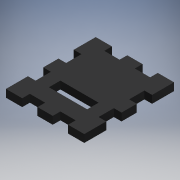
# Autodesk Inventor part: right
Saved by Autodesk Inventor 2019 (Build 230136000, 136)
## iProperties
Created: 2018-06-06
Part Number: right
Material: PBT Plastic Black
Document SubType Name: Modeling
Designer: stra92745
Density: 1.31 g/cm^3
Appearance: Smooth - White
Author: stra92745
Autodesk Inventor part; units mm, degrees
ref_plane "YZ Plane" through (0, 0, 0) normal (1, 0, 0) x (0, 1, 0)
ref_plane "XZ Plane" through (0, 0, 0) normal (0, 1, 0) x (-1, 0, 0)
ref_plane "XY Plane" through (0, 0, 0) normal (0, 0, 1) x (1, 0, 0)
sketch "Sketch1" plane through (0, 0, 0) normal (0, 1, 0) x (-1, 0, 0)
  line L0 (0, 0) -> (-41, 0)
  line L1 (-41, 0) -> (-41, -47)
  line L2 (-41, -47) -> (0, -47)
  line L3 (0, -47) -> (0, 0)
  line L4 (-10.5, -18) -> (-30.5, -18)
  line L5 (-30.5, -18) -> (-30.5, -12)
  line L6 (-30.5, -12) -> (-10.5, -12)
  line L7 (-10.5, -12) -> (-10.5, -18)
  dimension "d0" = 41
  dimension "d1" = 47
  dimension "d2" = 20
  dimension "d3" = 6
  dimension "d4" = 10.5
  dimension "d5" = 12
  constraints: 16 end point, 4 parallel, 2 horizontal, 2 perpendicular
  measures "d0" distance of L2.end L1.end
  measures "d1" distance of L1.end L0.end
  measures "d2" distance of L4.start L4.end
  measures "d3" distance of L4.end L5.end
  measures "d4" distance between parallel lines of L7 L3
  measures "d5" distance between parallel lines of L0 L6
extrude "Extrusion1" add sketch "Sketch1" along normal blind 4
sketch "Sketch2" plane through (0, 4, 0) normal (0, 1, 0) x (1, 0, 0)
  line L0 (41, 47) -> (0, 47) construction
  line L1 (0, 47) -> (0, 0) construction
  line L2 (0, 0) -> (41, 0) construction
  line L3 (41, 0) -> (41, 47) construction
  line L4 (4, 4) -> (4, 43) construction
  line L5 (4, 43) -> (37, 43) construction
  line L6 (37, 43) -> (37, 4) construction
  line L7 (37, 4) -> (4, 4) construction
  line L8 (0, 35.5) -> (4, 35.5)
  line L9 (4, 35.5) -> (4, 27.5)
  line L10 (4, 27.5) -> (0, 27.5)
  line L11 (0, 35.5) -> (0, 27.5)
  line L12 (0, 23.5) -> (41, 23.5) construction
  line L13 (20.5, 0) -> (20.5, 47) construction
  line L14 (41, 47) -> (0, 47) construction
  line L15 (8.5, 47) -> (8.5, 43)
  line L16 (8.5, 43) -> (16.5, 43)
  line L17 (16.5, 43) -> (16.5, 47)
  line L18 (16.5, 47) -> (8.5, 47)
  line L19 (41, 35.5) -> (37, 35.5)
  line L20 (37, 35.5) -> (37, 27.5)
  line L21 (37, 27.5) -> (41, 27.5)
  line L22 (41, 35.5) -> (41, 27.5)
  line L23 (32.5, 47) -> (32.5, 43)
  line L24 (32.5, 43) -> (24.5, 43)
  line L25 (24.5, 43) -> (24.5, 47)
  line L26 (24.5, 47) -> (32.5, 47)
  line L27 (41, 0) -> (0, 0)
  line L28 (4, 4) -> (37, 4)
  line L29 (0, 11.5) -> (4, 11.5)
  line L30 (4, 11.5) -> (4, 19.5)
  line L31 (4, 19.5) -> (0, 19.5)
  line L32 (0, 11.5) -> (0, 19.5)
  line L33 (41, 0) -> (0, 0)
  line L34 (8.5, 0) -> (8.5, 4)
  line L35 (8.5, 4) -> (16.5, 4)
  line L36 (16.5, 4) -> (16.5, 0)
  line L37 (16.5, 0) -> (8.5, 0)
  line L38 (24.5, 4) -> (24.5, 0)
  line L39 (32.5, 0) -> (32.5, 4)
  line L40 (37, 11.5) -> (37, 19.5)
  line L41 (41, 11.5) -> (37, 11.5)
  line L42 (41, 11.5) -> (41, 19.5)
  line L43 (37, 19.5) -> (41, 19.5)
  line L44 (24.5, 0) -> (32.5, 0)
  line L45 (32.5, 4) -> (24.5, 4)
  dimension "d8" = 4
  dimension "d9" = 8
  dimension "d10" = 4
  dimension "d11" = 8
  dimension "d12" = 4
  constraints: 82 end point, 24 symmetric about line, 12 point on line, 4 midpoint, 4 perpendicular, 2 collinear, 3 other
  measures "d8" distance between parallel lines of L1 L4
  measures "d9" distance of L8.end L9.end
  measures "d10" distance between parallel lines of L12 L10
  measures "d11" distance of L15.end L16.end
  measures "d12" distance between parallel lines of L13 L17
extrude "Extrusion2" cut sketch "Sketch2" against normal up to surface (4 mm away) contours L8 L9 L10 L11 | L18 L17 L16 L15 | L22 L21 L20 L19 | L23 L24 L25 L26 | L27 L38 L28 L39 | L27 L34 L28 L36 | L32 L31 L30 L29 | L40 L43 L42 L41
body "Solid1"
